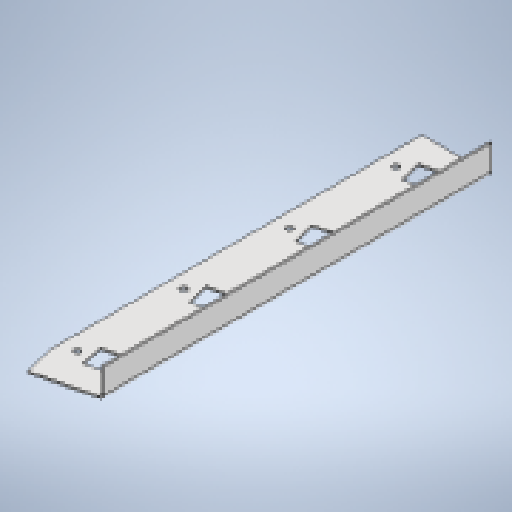
# Autodesk Inventor part: DS-B-103 Ridge top
Saved by Autodesk Inventor 2025 (Build 290162010, 162A)
## iProperties
Created: 2025-01-16
Part Number: DS-B-103 Ridge top
Material: Stainless Steel
Document SubType Name: Sheet Metal
Designer: pokla
Density: 8 g/cm^3
Sheet Metal Rule: AISI304 3mm Die 32
Appearance: Default
Flat Pattern Width: 14.3927 cm
Flat Pattern Length: 60.5365 cm
Flat Pattern Area: 871.286 cm^2
Sheet Metal Width: 143,927 mm
Sheet Metal Length: 605,365 mm
Sheet Metal Area: 87128,593 mm^2
Mass: 1289.63 g
Surface Area: 1660.36 cm^2
Volume: 161.204 cm^3
Author: pokla
Autodesk Inventor part; units mm, degrees
ref_plane "YZ Plane" through (0, 0, 0) normal (1, 0, 0) x (0, 1, 0)
ref_plane "XZ Plane" through (0, 0, 0) normal (0, 1, 0) x (-1, 0, 0)
ref_plane "XY Plane" through (0, 0, 0) normal (0, 0, 1) x (1, 0, 0)
sketch "Sketch1" plane through (0, 0, 0) normal (0, 0, 1) x (1, 0, 0)
  line L0 (-52.5, 292) -> (52.5, 292)
  line L1 (52.5, 292) -> (52.5, -292)
  line L2 (52.5, -292) -> (-52.5, -292)
  line L3 (-52.5, -292) -> (-52.5, 292)
  line L4 (-52.5, 292) -> (52.5, -292) construction
  point P0 (0, 0)
  point P1 (0, 0)
  dimension "d0" = 105
  dimension "d1" = 584
  measures "d0" distance of L0.start L0.end
  measures "d1" distance of L2.end L0.start
extrude "Plate1" add sketch "Sketch1" along normal blind 3
sketch "Sketch4" plane through (49.5, 292, 0) normal (1, 0, 0) x (0, 1, 0)
  line L0 (-584, 0) -> (0, 0)
  line L1 (0, 0) -> (0, 45)
  line L2 (0, 45) -> (-584, 45)
  line L3 (-584, 45) -> (-584, 0)
  constraints: 6 end point, 1 horizontal, 1 perpendicular, 1 vertical
edge flange "Flange1" height 45 angle 90 thickness 3 bend radius 5 thickness toward (1, 0, 0) relief round relief width 3 relief depth 1.5 edges at (52.5, 0, 3) wall of the first edge with corners at (49.5, -292, 0) (49.5, 292, 0) (49.5, 292, 45) (49.5, -292, 45)
bend "Bend1"
corner "Corner1"
sketch "Sketch5" plane through (0, 0, 0) normal (0, 0, -1) x (-1, 0, 0)
  line L0 (-44.5, 292) -> (-44.5, -292) projected
  line L1 (52.5, -292) -> (-44.5, -292) projected
  line L2 (52.5, 292) -> (52.5, -292) projected
  line L3 (-44.5, 292) -> (52.5, 292) projected
  line L4 (52.5, -292) -> (52.5, -316.1848)
  line L5 (-44.5, -292) -> (52.5, -292) projected
  line L6 (52.5, -316.1848) -> (-44.5, -292)
  point P0 (0, 0)
  dimension "d25" = 14
  constraints: 4 end point, 1 vertical
  measures "d25" angle of L1 L6
extrude "Extrusion2" add sketch "Sketch5" against normal up to surface (3 mm away) contours L1 L4 L6
sketch "Sketch6" plane through (0, 0, 0) normal (0, 0, -1) x (-1, 0, 0)
  line L0 (-44.5, 292) -> (-44.5, -292) construction
  line L1 (-44.5, -292) -> (52.5, -316.1848) projected
  line L2 (52.5, 292) -> (52.5, -316.1848) projected
  line L3 (-44.5, 292) -> (52.5, 292) construction
  line L4 (41.1893, -313.3647) -> (52.5, -268)
  line L5 (-44.5, -292) -> (52.5, -316.1848) projected
  point P0 (0, 0)
  dimension "d45" = 560
  constraints: 2 end point, 2 point on line, 1 perpendicular
  measures "d45" distance from line of L3 L4.end
extrude "Cut1" cut sketch "Sketch6" against normal blind 3
sketch "Sketch7" plane through (0, 0, 0) normal (0, 0, 1) x (1, 0, 0)
  line L0 (44.5, -292) -> (-41.1893, -313.3647) projected
  circle A0 centre (36.1472, -268.8326) radius 5.05
  line L1 (36.1472, -268.8326) -> (19.2126, -200.9119) construction
  line L2 (24.6363, -253.6668) -> (16.1691, -219.7064)
  circle A1 centre (19.2126, -200.9119) radius 5.05
  line L3 (-30.5378, -249.3875) -> (36.1472, -268.8326) construction
  line L4 (24.6363, -253.6668) -> (-17.7913, -228.1737) construction
  line L5 (16.1691, -219.7064) -> (-17.7913, -228.1737)
  line L6 (-9.324, -262.1341) -> (24.6363, -253.6668)
  line L7 (16.1691, -219.7064) -> (-9.324, -262.1341) construction
  line L8 (-17.7913, -228.1737) -> (-9.324, -262.1341)
  line L9 (20.4027, -236.6866) -> (-30.5378, -249.3875) construction
  line L10 (19.2126, -200.9119) -> (-30.5378, -249.3875) construction
  circle A2 centre (-30.5378, -249.3875) radius 5.05
  point P0 (0, 0)
  point P1 (3.4225, -240.9203)
  dimension "d32" = 35
  dimension "d33" = 35
  dimension "d34" = 10.1
  dimension "d35" = 70
  dimension "d36" = 60
  dimension "d37" = 25
  dimension "d38" = 10
  dimension "d39" = 42
  constraints: 20 end point, 3 centre point, 3 midpoint, 3 parallel, 2 perpendicular, 1 equal radius, 2 other
  measures "d32" distance of L6.start L4.end
  measures "d33" distance of L4.end L2.end
  measures "d34" diameter of A2
  measures "d35" distance of L1.start L1.end
  measures "d36" distance from line of L3.start L1
  measures "d37" distance from line of L1 point (3.423, -240.92)
  measures "d38" distance from line of L0.start L2
  measures "d39" distance between parallel lines of L0 L6
extrude "Extrusion3" cut sketch "Sketch7" along normal through all
pattern_linear "Rectangular Pattern1" count 4 spacing 160 along (0, 1, 0) of "Extrusion3"
equation "\"d0\" = RIDGE_1_hight"
equation "\"d25\" = RIDGE_1_angle"
equation "\"d45\" = RIDGE_1_lenth"
equation "\"d30\" = Thickness"
equation "\"d33\" = d32"
equation "\"d2\" = Thickness"
equation "\"d15\" = BendReliefWidth"
equation "\"d16\" = BendReliefDepth"
equation "\"d17\" = MinimumRemnant"
equation "\"d18\" = TransitionRadius"
equation "\"d21\" = BendRadius"
equation "\"d22\" = CornerReliefSize"
equation "\"d23\" = GapSize"
equation "\"d24\" = JacobiRadiusSize"
equation "\"BendReliefWidth\" = Thickness"
equation "\"BendReliefDepth\" = 0.5 * Thickness"
equation "\"CornerReliefSize\" = 4 * Thickness"
equation "\"MinimumRemnant\" = 2 * Thickness"
equation "\"TransitionRadius\" = BendRadius"
equation "\"JacobiRadiusSize\" = BendRadius"
equation "\"GapSize\" = Thickness"
equation "\"RIDGE_1_hight\" = 105"
equation "\"RIDGE_1_angle\" = 14deg"
equation "\"RIDGE_1_lenth\" = 560"
equation "\"Thickness\" = 3"
equation "\"BendRadius\" = 5"
body "Solid1"
